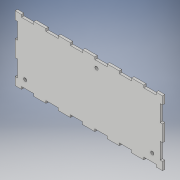
# Autodesk Inventor part: 12 boven plaat LCD
Saved by Autodesk Inventor 2019 (Build 230136000, 136)
## iProperties
Created: 2021-04-20
Part Number: 12 boven plaat LCD
Material: Generic
Document SubType Name: Sheet Metal
Designer: Stefan
Density: 1 g/cm^3
Sheet Metal Rule: Default_mm
Appearance: Default
Author: Stefan
Autodesk Inventor part; units mm, degrees
ref_plane "YZ Plane" through (0, 0, 0) normal (1, 0, 0) x (0, 1, 0)
ref_plane "XZ Plane" through (0, 0, 0) normal (0, 1, 0) x (-1, 0, 0)
ref_plane "XY Plane" through (0, 0, 0) normal (0, 0, 1) x (1, 0, 0)
sketch "Sketch1" plane through (0, 0, 0) normal (0, 0, 1) x (1, 0, 0)
  line L0 (-87.5, -36.75) -> (87.5, -36.75)
  line L1 (87.5, -36.75) -> (87.5, 36.75)
  line L2 (87.5, 36.75) -> (-87.5, 36.75)
  line L3 (-87.5, 36.75) -> (-87.5, -36.75)
  line L4 (-87.5, -36.75) -> (87.5, 36.75) construction
  line L5 (87.5, -36.75) -> (-87.5, 36.75) construction
  line L6 (-67.5, 36.75) -> (-52.5, 36.75)
  line L7 (-52.5, 36.75) -> (-52.5, 39.75)
  line L8 (-52.5, 39.75) -> (-67.5, 39.75)
  line L9 (-67.5, 39.75) -> (-67.5, 36.75)
  line L10 (-87.5, 10) -> (-90.5, 10)
  line L11 (-90.5, 10) -> (-90.5, -10)
  line L12 (-90.5, -10) -> (-87.5, -10)
  line L13 (-87.5, -10) -> (-87.5, 10)
  line L14 (-82.5, 36.75) -> (-82.5, 39.75)
  line L15 (-87.5, 30) -> (-90.5, 30)
  line L16 (-90.5, 30) -> (-90.5, 39.75)
  line L17 (-90.5, 39.75) -> (-82.5, 39.75)
  line L18 (-22.5, 36.75) -> (-22.5, 39.75)
  line L19 (-22.5, 39.75) -> (-37.5, 39.75)
  line L20 (-37.5, 39.75) -> (-37.5, 36.75)
  line L21 (-37.5, 36.75) -> (-22.5, 36.75)
  line L22 (7.5, 36.75) -> (7.5, 39.75)
  line L23 (7.5, 39.75) -> (-7.5, 39.75)
  line L24 (-7.5, 39.75) -> (-7.5, 36.75)
  line L25 (-7.5, 36.75) -> (7.5, 36.75)
  line L26 (37.5, 36.75) -> (37.5, 39.75)
  line L27 (37.5, 39.75) -> (22.5, 39.75)
  line L28 (22.5, 39.75) -> (22.5, 36.75)
  line L29 (22.5, 36.75) -> (37.5, 36.75)
  line L30 (67.5, 36.75) -> (67.5, 39.75)
  line L31 (67.5, 39.75) -> (52.5, 39.75)
  line L32 (52.5, 39.75) -> (52.5, 36.75)
  line L33 (52.5, 36.75) -> (67.5, 36.75)
  line L34 (-52.5, -39.75) -> (-52.5, -36.75)
  line L35 (-52.5, -36.75) -> (-67.5, -36.75)
  line L36 (-67.5, -36.75) -> (-67.5, -39.75)
  line L37 (-67.5, -39.75) -> (-52.5, -39.75)
  line L38 (-22.5, -39.75) -> (-22.5, -36.75)
  line L39 (-22.5, -36.75) -> (-37.5, -36.75)
  line L40 (-37.5, -36.75) -> (-37.5, -39.75)
  line L41 (-37.5, -39.75) -> (-22.5, -39.75)
  line L42 (7.5, -39.75) -> (7.5, -36.75)
  line L43 (7.5, -36.75) -> (-7.5, -36.75)
  line L44 (-7.5, -36.75) -> (-7.5, -39.75)
  line L45 (-7.5, -39.75) -> (7.5, -39.75)
  line L46 (37.5, -39.75) -> (37.5, -36.75)
  line L47 (37.5, -36.75) -> (22.5, -36.75)
  line L48 (22.5, -36.75) -> (22.5, -39.75)
  line L49 (22.5, -39.75) -> (37.5, -39.75)
  line L50 (67.5, -39.75) -> (67.5, -36.75)
  line L51 (67.5, -36.75) -> (52.5, -36.75)
  line L52 (52.5, -36.75) -> (52.5, -39.75)
  line L53 (52.5, -39.75) -> (67.5, -39.75)
  line L54 (90.5, 10) -> (87.5, 10)
  line L55 (87.5, 10) -> (87.5, -10)
  line L56 (87.5, -10) -> (90.5, -10)
  line L57 (90.5, -10) -> (90.5, 10)
  line L58 (-87.5, 0) -> (87.5, 0) construction
  line L59 (0, 36.75) -> (0, -36.75) construction
  line L60 (-87.5, 30) -> (-87.5, 36.75)
  line L61 (-82.5, 36.75) -> (-87.5, 36.75)
  line L62 (-82.5, -36.75) -> (-82.5, -39.75)
  line L63 (-87.5, -30) -> (-90.5, -30)
  line L64 (-90.5, -30) -> (-90.5, -39.75)
  line L65 (-90.5, -39.75) -> (-82.5, -39.75)
  line L66 (-87.5, -30) -> (-87.5, -36.75)
  line L67 (-82.5, -36.75) -> (-87.5, -36.75)
  line L68 (82.5, 36.75) -> (82.5, 39.75)
  line L69 (87.5, 30) -> (90.5, 30)
  line L70 (90.5, 30) -> (90.5, 39.75)
  line L71 (90.5, 39.75) -> (82.5, 39.75)
  line L72 (87.5, 30) -> (87.5, 36.75)
  line L73 (82.5, 36.75) -> (87.5, 36.75)
  line L74 (82.5, -36.75) -> (82.5, -39.75)
  line L75 (87.5, -30) -> (90.5, -30)
  line L76 (90.5, -30) -> (90.5, -39.75)
  line L77 (90.5, -39.75) -> (82.5, -39.75)
  line L78 (87.5, -30) -> (87.5, -36.75)
  line L79 (82.5, -36.75) -> (87.5, -36.75)
  point P0 (0, 0)
  dimension "d0" = 175
  dimension "d1" = 73.5
  dimension "d2" = 15
  dimension "d3" = 3
  dimension "d4" = 20
  dimension "d5" = 3
  dimension "d6" = 20
  dimension "d7" = 10
  dimension "d8" = 3
  dimension "d9" = 15
  dimension "d10" = 3
  dimension "d11" = 20
  dimension "d14" = 30
  dimension "d17" = 76.5
  dimension "d22" = 178
  constraints: 160 end point, 15 symmetric about line, 6 horizontal, 6 midpoint, 6 parallel, 5 perpendicular, 4 point on line, 3 vertical, 1 collinear, 80 other
  measures "d0" distance of L2.end L1.end
  measures "d1" distance of L1.end L0.end
  measures "d2" distance of L8.end L7.end
  measures "d3" distance of L7.end L6.end
  measures "d4" distance between parallel lines of L9 L3
  measures "d5" distance of L12.end L11.end
  measures "d6" distance of L11.end L10.end
  measures "d7" distance from line of point (0, 0) L10
  measures "d8" distance of L14.start L14.end
  measures "d9" distance between parallel lines of L9 L14
  measures "d10" distance of L15.start L15.end
  measures "d11" distance between parallel lines of L15 L10
  measures "d14" distance of L7.end L18.end
  measures "d17" distance of L7.end L34.end
  measures "d22" distance of L10.start L54.start
extrude "Extrusion1" add sketch "Sketch1" along normal blind 3
sketch "Sketch2" plane through (0, 0, 3) normal (0, 0, 1) x (1, 0, 0)
  circle A0 centre (-78, -27.25) radius 2
  circle A1 centre (78, -27.25) radius 2
  line L0 (87.5, -30) -> (87.5, -10) projected
  line L1 (67.5, -36.75) -> (82.5, -36.75) projected
  line L2 (-82.5, -36.75) -> (-67.5, -36.75) projected
  line L3 (-87.5, -10) -> (-87.5, -30) projected
  point P0 (0, 0)
  dimension "d29" = 4
  dimension "d30" = 4
  dimension "d31" = 9.5
  dimension "d32" = 9.5
  dimension "d33" = 9.5
  dimension "d34" = 9.5
  constraints: 2 centre point
  measures "d29" diameter of A0
  measures "d30" diameter of A1
  measures "d31" distance from line of L0 A1.centre
  measures "d32" distance from line of L1 A1.centre
  measures "d33" distance from line of L2 A0.centre
  measures "d34" distance from line of A0.centre L3
extrude "Extrusion2" cut sketch "Sketch2" against normal blind 10
sketch "Sketch3" plane through (0, 0, 0) normal (0, 0, -1) x (-1, 0, 0)
  circle A0 centre (-9.5, 28.75) radius 2
  line L0 (-7.5, 39.75) -> (-7.5, 36.75) projected
  line L1 (-22.5, 36.75) -> (-7.5, 36.75) projected
  point P0 (0, 0)
  dimension "d37" = 4
  dimension "d38" = 2
  dimension "d39" = 8
  constraints: 1 centre point
  measures "d37" diameter of A0
  measures "d38" distance from line of A0.centre L0
  measures "d39" distance from line of L1 A0.centre
extrude "Extrusion3" cut sketch "Sketch3" against normal blind 10
equation "\"BendRadius\" = Thickness"
equation "\"BendReliefWidth\" = Thickness"
equation "\"BendReliefDepth\" = 0.5 * Thickness"
equation "\"CornerReliefSize\" = 4 * Thickness"
equation "\"MinimumRemnant\" = 2 * Thickness"
equation "\"TransitionRadius\" = BendRadius"
equation "\"JacobiRadiusSize\" = BendRadius"
equation "\"GapSize\" = Thickness"
equation "\"Thickness\" = 0.5"
body "Solid1"
